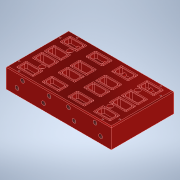
# Autodesk Inventor part: UNLHEP-14-01-P-004_ChuckForGantry
Saved by Autodesk Inventor 2022 (Build 260153000, 153)
## iProperties
Created: 2014-01-09
Part Number: UNLHEP-14-01-P-004_ChuckForGantry
Material: Aluminum, Anodized Red
Document SubType Name: Modeling
Designer: Frank Meier
Density: 2.7 g/cm^3
Project: UNL Pixel Phase I
Mass: 2699.72 g
Surface Area: 1115.91 cm^2
Volume: 999.896 cm^3
Appearance: Anodized - Red
Author: Frank Meier
Revision Number: 00
Autodesk Inventor part; units mm, degrees
ref_plane "YZ Plane" through (0, 0, 0) normal (1, 0, 0) x (0, 1, 0)
ref_plane "XZ Plane" through (0, 0, 0) normal (0, 1, 0) x (-1, 0, 0)
ref_plane "XY Plane" through (0, 0, 0) normal (0, 0, 1) x (1, 0, 0)
sketch "Skizze1" plane through (0, 0, 0) normal (0, 0, 1) x (1, 0, 0)
  line L0 (-117.475, -69.85) -> (117.475, -69.85)
  line L1 (117.475, -69.85) -> (117.475, 69.85)
  line L2 (117.475, 69.85) -> (-117.475, 69.85)
  line L3 (-117.475, 69.85) -> (-117.475, -69.85)
  line L4 (-117.475, -69.85) -> (117.475, 69.85) construction
  line L5 (117.475, -69.85) -> (-117.475, 69.85) construction
  point P0 (0, 0)
  dimension "d0" = 234.95
  dimension "d2" = 139.7
  constraints: 12 end point, 2 midpoint, 2 parallel, 1 horizontal, 1 perpendicular
  measures "d0" distance of L1.end L2.end
  measures "d2" distance of L0.end L1.end
extrude "Extrusion1" add sketch "Skizze1" along normal blind 44.45
chamfer "Fase1" distance 2 angle 45 4 edges at (0, -69.85, 44.45) (-117.475, 0, 44.45) (0, 69.85, 44.45) (117.475, 0, 44.45)
sketch "Alignment Holes" plane through (0, 0, 44.45) normal (0, 0, 1) x (1, 0, 0)
  line L0 (117.475, 69.85) -> (-117.475, 69.85) projected
  line L1 (117.475, -69.85) -> (117.475, 69.85) projected
  line L2 (-117.475, 69.85) -> (-117.475, -69.85) projected
  line L3 (-117.475, -69.85) -> (117.475, -69.85) projected
  point P0 (-112.475, 45.85)
  point P1 (-112.475, -45.85)
  point P2 (-93.475, -64.85)
  point P3 (-93.475, 64.85)
  point P4 (93.475, 64.85)
  point P5 (112.475, 45.85)
  point P6 (112.475, -45.85)
  point P7 (93.475, -64.85)
  dimension "d153" = 24
  dimension "d154" = 24
  dimension "d155" = 5
  dimension "d156" = 5
  dimension "d157" = 24
  dimension "d158" = 5
  dimension "d159" = 5
  dimension "d160" = 24
  dimension "d161" = 24
  dimension "d162" = 5
  dimension "d163" = 5
  dimension "d164" = 24
  dimension "d165" = 5
  dimension "d166" = 24
  dimension "d167" = 5
  dimension "d168" = 24
  measures "d153" distance from line of L0 point (-112.475, 45.85)
  measures "d154" distance from line of L3 point (-112.475, -45.85)
  measures "d155" distance from line of L2 point (-112.475, -45.85)
  measures "d156" distance from line of L3 point (-93.475, -64.85)
  measures "d157" distance from line of L2 point (-93.475, -64.85)
  measures "d158" distance from line of L2 point (-112.475, 45.85)
  measures "d159" distance from line of L0 point (-93.475, 64.85)
  measures "d160" distance from line of L2 point (-93.475, 64.85)
  measures "d161" distance from line of L1 point (93.475, 64.85)
  measures "d162" distance from line of L0 point (93.475, 64.85)
  measures "d163" distance from line of L1 point (112.475, 45.85)
  measures "d164" distance from line of L0 point (112.475, 45.85)
  measures "d165" distance from line of L1 point (112.475, -45.85)
  measures "d166" distance from line of L3 point (112.475, -45.85)
  measures "d167" distance from line of L3 point (93.475, -64.85)
  measures "d168" distance from line of L1 point (93.475, -64.85)
hole "Bohrung7" at (-112.475, 45.85, 44.45) at (-112.475, -45.85, 44.45) at (-93.475, -64.85, 44.45) at (-93.475, 64.85, 44.45) at (93.475, 64.85, 44.45) at (112.475, 45.85, 44.45) at (112.475, -45.85, 44.45) at (93.475, -64.85, 44.45) direction (0, 0, -1) diameter 3.242 depth 20 tip angle 118 thread size "M4x0.7" class "6H" standard "ISO Metric profile"
sketch "Wells" plane through (0, 0, 44.45) normal (0, 0, 1) x (1, 0, 0)
  line L0 (-97.975, 56.35) -> (-73.975, 56.35)
  line L1 (-70.975, 53.35) -> (-70.975, 44.35)
  line L2 (-73.975, 41.35) -> (-97.975, 41.35)
  line L3 (-100.975, 44.35) -> (-100.975, 53.35)
  circle A0 centre (-93.475, 64.85) radius 1.621 projected
  circle A1 centre (-112.475, 45.85) radius 1.621 projected
  arc A2 (-97.975, 56.35) -> (-100.975, 53.35) centre (-97.975, 53.35) ccw
  arc A3 (-70.975, 53.35) -> (-73.975, 56.35) centre (-73.975, 53.35) ccw
  arc A4 (-73.975, 41.35) -> (-70.975, 44.35) centre (-73.975, 44.35) ccw
  arc A5 (-100.975, 44.35) -> (-97.975, 41.35) centre (-97.975, 44.35) ccw
  arc A6 (-40.658, 56.35) -> (-43.658, 53.35) centre (-40.658, 53.35) ccw
  line L4 (-43.658, 44.35) -> (-43.658, 53.35)
  arc A7 (-43.658, 44.35) -> (-40.658, 41.35) centre (-40.658, 44.35) ccw
  line L5 (-40.658, 56.35) -> (-16.658, 56.35)
  arc A8 (-13.658, 53.35) -> (-16.658, 56.35) centre (-16.658, 53.35) ccw
  line L6 (-13.658, 53.35) -> (-13.658, 44.35)
  line L7 (-16.658, 41.35) -> (-40.658, 41.35)
  arc A9 (-16.658, 41.35) -> (-13.658, 44.35) centre (-16.658, 44.35) ccw
  arc A10 (16.659, 56.35) -> (13.659, 53.35) centre (16.659, 53.35) ccw
  line L8 (13.659, 44.35) -> (13.659, 53.35)
  arc A11 (13.659, 44.35) -> (16.659, 41.35) centre (16.659, 44.35) ccw
  line L9 (16.659, 56.35) -> (40.659, 56.35)
  arc A12 (43.659, 53.35) -> (40.659, 56.35) centre (40.659, 53.35) ccw
  line L10 (43.659, 53.35) -> (43.659, 44.35)
  line L11 (40.659, 41.35) -> (16.659, 41.35)
  arc A13 (40.659, 41.35) -> (43.659, 44.35) centre (40.659, 44.35) ccw
  arc A14 (73.976, 56.35) -> (70.976, 53.35) centre (73.976, 53.35) ccw
  line L12 (70.976, 44.35) -> (70.976, 53.35)
  arc A15 (70.976, 44.35) -> (73.976, 41.35) centre (73.976, 44.35) ccw
  line L13 (73.976, 56.35) -> (97.976, 56.35)
  arc A16 (100.976, 53.35) -> (97.976, 56.35) centre (97.976, 53.35) ccw
  line L14 (100.976, 53.35) -> (100.976, 44.35)
  line L15 (97.976, 41.35) -> (73.976, 41.35)
  arc A17 (97.976, 41.35) -> (100.976, 44.35) centre (97.976, 44.35) ccw
  arc A18 (-97.975, 20.784) -> (-100.975, 17.784) centre (-97.975, 17.784) ccw
  line L16 (-100.975, 8.784) -> (-100.975, 17.784)
  arc A19 (-100.975, 8.784) -> (-97.975, 5.784) centre (-97.975, 8.784) ccw
  line L17 (-97.975, 20.784) -> (-73.975, 20.784)
  arc A20 (-70.975, 17.784) -> (-73.975, 20.784) centre (-73.975, 17.784) ccw
  line L18 (-70.975, 17.784) -> (-70.975, 8.784)
  line L19 (-73.975, 5.784) -> (-97.975, 5.784)
  arc A21 (-73.975, 5.784) -> (-70.975, 8.784) centre (-73.975, 8.784) ccw
  arc A22 (-40.658, 20.784) -> (-43.658, 17.784) centre (-40.658, 17.784) ccw
  line L20 (-43.658, 8.784) -> (-43.658, 17.784)
  arc A23 (-43.658, 8.784) -> (-40.658, 5.784) centre (-40.658, 8.784) ccw
  line L21 (-40.658, 20.784) -> (-16.658, 20.784)
  arc A24 (-13.658, 17.784) -> (-16.658, 20.784) centre (-16.658, 17.784) ccw
  line L22 (-13.658, 17.784) -> (-13.658, 8.784)
  line L23 (-16.658, 5.784) -> (-40.658, 5.784)
  arc A25 (-16.658, 5.784) -> (-13.658, 8.784) centre (-16.658, 8.784) ccw
  arc A26 (16.659, 20.784) -> (13.659, 17.784) centre (16.659, 17.784) ccw
  line L24 (13.659, 8.784) -> (13.659, 17.784)
  arc A27 (13.659, 8.784) -> (16.659, 5.784) centre (16.659, 8.784) ccw
  line L25 (16.659, 20.784) -> (40.659, 20.784)
  arc A28 (43.659, 17.784) -> (40.659, 20.784) centre (40.659, 17.784) ccw
  line L26 (43.659, 17.784) -> (43.659, 8.784)
  line L27 (40.659, 5.784) -> (16.659, 5.784)
  arc A29 (40.659, 5.784) -> (43.659, 8.784) centre (40.659, 8.784) ccw
  arc A30 (73.976, 20.784) -> (70.976, 17.784) centre (73.976, 17.784) ccw
  line L28 (70.976, 8.784) -> (70.976, 17.784)
  arc A31 (70.976, 8.784) -> (73.976, 5.784) centre (73.976, 8.784) ccw
  line L29 (73.976, 20.784) -> (97.976, 20.784)
  arc A32 (100.976, 17.784) -> (97.976, 20.784) centre (97.976, 17.784) ccw
  line L30 (100.976, 17.784) -> (100.976, 8.784)
  line L31 (97.976, 5.784) -> (73.976, 5.784)
  arc A33 (97.976, 5.784) -> (100.976, 8.784) centre (97.976, 8.784) ccw
  circle A34 centre (-93.475, -64.85) radius 1.621 projected
  circle A35 centre (112.475, 45.85) radius 1.621 projected
  line L32 (97.975, -56.35) -> (73.975, -56.35)
  line L33 (70.975, -53.35) -> (70.975, -44.35)
  line L34 (73.975, -41.35) -> (97.975, -41.35)
  line L35 (100.975, -44.35) -> (100.975, -53.35)
  circle A36 centre (112.475, -45.85) radius 1.621 projected
  circle A37 centre (93.475, -64.85) radius 1.621 projected
  arc A38 (73.975, -41.35) -> (70.975, -44.35) centre (73.975, -44.35) ccw
  arc A39 (70.975, -53.35) -> (73.975, -56.35) centre (73.975, -53.35) ccw
  arc A40 (97.975, -56.35) -> (100.975, -53.35) centre (97.975, -53.35) ccw
  arc A41 (100.975, -44.35) -> (97.975, -41.35) centre (97.975, -44.35) ccw
  arc A42 (43.658, -44.35) -> (40.658, -41.35) centre (40.658, -44.35) ccw
  line L36 (16.658, -41.35) -> (40.658, -41.35)
  line L37 (43.658, -44.35) -> (43.658, -53.35)
  arc A43 (40.658, -56.35) -> (43.658, -53.35) centre (40.658, -53.35) ccw
  line L38 (40.658, -56.35) -> (16.658, -56.35)
  arc A44 (16.658, -41.35) -> (13.658, -44.35) centre (16.658, -44.35) ccw
  arc A45 (13.658, -53.35) -> (16.658, -56.35) centre (16.658, -53.35) ccw
  line L39 (13.658, -53.35) -> (13.658, -44.35)
  arc A46 (-13.659, -44.35) -> (-16.659, -41.35) centre (-16.659, -44.35) ccw
  line L40 (-40.659, -41.35) -> (-16.659, -41.35)
  line L41 (-13.659, -44.35) -> (-13.659, -53.35)
  arc A47 (-16.659, -56.35) -> (-13.659, -53.35) centre (-16.659, -53.35) ccw
  line L42 (-16.659, -56.35) -> (-40.659, -56.35)
  arc A48 (-40.659, -41.35) -> (-43.659, -44.35) centre (-40.659, -44.35) ccw
  arc A49 (-43.659, -53.35) -> (-40.659, -56.35) centre (-40.659, -53.35) ccw
  line L43 (-43.659, -53.35) -> (-43.659, -44.35)
  arc A50 (-70.976, -44.35) -> (-73.976, -41.35) centre (-73.976, -44.35) ccw
  line L44 (-97.976, -41.35) -> (-73.976, -41.35)
  line L45 (-70.976, -44.35) -> (-70.976, -53.35)
  arc A51 (-73.976, -56.35) -> (-70.976, -53.35) centre (-73.976, -53.35) ccw
  line L46 (-73.976, -56.35) -> (-97.976, -56.35)
  arc A52 (-97.976, -41.35) -> (-100.976, -44.35) centre (-97.976, -44.35) ccw
  arc A53 (-100.976, -53.35) -> (-97.976, -56.35) centre (-97.976, -53.35) ccw
  line L47 (-100.976, -53.35) -> (-100.976, -44.35)
  arc A54 (100.975, -8.784) -> (97.975, -5.784) centre (97.975, -8.784) ccw
  line L48 (73.975, -5.784) -> (97.975, -5.784)
  line L49 (100.975, -8.784) -> (100.975, -17.784)
  arc A55 (97.975, -20.784) -> (100.975, -17.784) centre (97.975, -17.784) ccw
  line L50 (97.975, -20.784) -> (73.975, -20.784)
  arc A56 (73.975, -5.784) -> (70.975, -8.784) centre (73.975, -8.784) ccw
  arc A57 (70.975, -17.784) -> (73.975, -20.784) centre (73.975, -17.784) ccw
  line L51 (70.975, -17.784) -> (70.975, -8.784)
  arc A58 (43.658, -8.784) -> (40.658, -5.784) centre (40.658, -8.784) ccw
  line L52 (16.658, -5.784) -> (40.658, -5.784)
  line L53 (43.658, -8.784) -> (43.658, -17.784)
  arc A59 (40.658, -20.784) -> (43.658, -17.784) centre (40.658, -17.784) ccw
  line L54 (40.658, -20.784) -> (16.658, -20.784)
  arc A60 (16.658, -5.784) -> (13.658, -8.784) centre (16.658, -8.784) ccw
  arc A61 (13.658, -17.784) -> (16.658, -20.784) centre (16.658, -17.784) ccw
  line L55 (13.658, -17.784) -> (13.658, -8.784)
  arc A62 (-13.659, -8.784) -> (-16.659, -5.784) centre (-16.659, -8.784) ccw
  line L56 (-40.659, -5.784) -> (-16.659, -5.784)
  line L57 (-13.659, -8.784) -> (-13.659, -17.784)
  arc A63 (-16.659, -20.784) -> (-13.659, -17.784) centre (-16.659, -17.784) ccw
  line L58 (-16.659, -20.784) -> (-40.659, -20.784)
  arc A64 (-40.659, -5.784) -> (-43.659, -8.784) centre (-40.659, -8.784) ccw
  arc A65 (-43.659, -17.784) -> (-40.659, -20.784) centre (-40.659, -17.784) ccw
  line L59 (-43.659, -17.784) -> (-43.659, -8.784)
  arc A66 (-70.976, -8.784) -> (-73.976, -5.784) centre (-73.976, -8.784) ccw
  line L60 (-97.976, -5.784) -> (-73.976, -5.784)
  line L61 (-70.976, -8.784) -> (-70.976, -17.784)
  arc A67 (-73.976, -20.784) -> (-70.976, -17.784) centre (-73.976, -17.784) ccw
  line L62 (-73.976, -20.784) -> (-97.976, -20.784)
  arc A68 (-97.976, -5.784) -> (-100.976, -8.784) centre (-97.976, -8.784) ccw
  arc A69 (-100.976, -17.784) -> (-97.976, -20.784) centre (-97.976, -17.784) ccw
  line L63 (-100.976, -17.784) -> (-100.976, -8.784)
  point P0 (0, 0)
  point P1 (-70.975, 41.35)
  point P2 (-70.975, 56.35)
  point P3 (-100.975, 41.35)
  point P4 (-43.658, 41.35)
  point P5 (-13.658, 56.35)
  point P6 (-13.658, 41.35)
  point P7 (13.659, 41.35)
  point P8 (43.659, 56.35)
  point P9 (43.659, 41.35)
  point P10 (70.976, 41.35)
  point P11 (100.976, 56.35)
  point P12 (100.976, 41.35)
  point P13 (-100.975, 5.784)
  point P14 (-70.975, 20.784)
  point P15 (-70.975, 5.784)
  point P16 (-43.658, 5.784)
  point P17 (-13.658, 20.784)
  point P18 (-13.658, 5.784)
  point P19 (13.659, 5.784)
  point P20 (43.659, 20.784)
  point P21 (43.659, 5.784)
  point P22 (70.976, 5.784)
  point P23 (100.976, 20.784)
  point P24 (100.976, 5.784)
  point P25 (100.975, -56.35)
  point P26 (70.975, -56.35)
  point P27 (100.975, -41.35)
  point P28 (43.658, -41.35)
  point P29 (43.658, -56.35)
  point P30 (13.658, -56.35)
  point P31 (-13.659, -41.35)
  point P32 (-13.659, -56.35)
  point P33 (-43.659, -56.35)
  point P34 (-70.976, -41.35)
  point P35 (-70.976, -56.35)
  point P36 (-100.976, -56.35)
  point P37 (100.975, -5.784)
  point P38 (100.975, -20.784)
  point P39 (70.975, -20.784)
  point P40 (43.658, -5.784)
  point P41 (43.658, -20.784)
  point P42 (13.658, -20.784)
  point P43 (-13.659, -5.784)
  point P44 (-13.659, -20.784)
  point P45 (-43.659, -20.784)
  point P46 (-70.976, -5.784)
  point P47 (-70.976, -20.784)
  point P48 (-100.976, -20.784)
  dimension "d259" = 30
  dimension "d260" = 15
  dimension "d261" = 8.5
  dimension "d262" = 11.5
  dimension "d266" = 3
  dimension "d269" = 57.317
  dimension "d272" = 35.566
  dimension "d276" = 11.499
  dimension "d410" = 11.5
  dimension "d411" = 8.5
  dimension "d412" = 15
  dimension "d413" = 30
  dimension "d414" = 3
  dimension "d417" = 57.317
  dimension "d420" = 35.566
  constraints: 128 end point, 128 point on circle, 96 point on line, 64 centre point, 16 tangent, 6 equal radius, 4 collinear, 4 horizontal, 4 parallel, 2 perpendicular, 2 vertical, 318 other
  measures "d259" distance of point (-70.975, 41.35) point (-100.975, 41.35)
  measures "d260" distance of point (-70.975, 56.35) point (-70.975, 41.35)
  measures "d261" distance from line of L0 A0.centre
  measures "d262" distance from line of L3 A1.centre
  measures "d266" radius of A2
  measures "d269" distance of L3.end L4.end
  measures "d272" distance of L3.end L16.end
  measures "d276" distance from line of L14 A35.centre
  measures "d410" distance from line of L35 A36.centre
  measures "d411" distance from line of A37.centre L32
  measures "d412" distance of point (100.975, -41.35) point (100.975, -56.35)
  measures "d413" distance of point (100.975, -56.35) point (70.975, -56.35)
  measures "d414" radius of A38
  measures "d417" distance of point (100.975, -41.35) point (43.658, -41.35)
  measures "d420" distance of point (100.975, -41.35) point (100.975, -5.784)
extrude "Extrusion6" cut sketch "Wells" against normal blind 10 contours L0 A3 L1 A4 L2 A5 L3 A2 | L5 A8 L6 A9 L7 A7 L4 A6 | L9 A12 L10 A13 L11 A11 L8 A10 | L13 A16 L14 A17 L15 A15 L12 A14 | L32 A39 L33 A38 L34 A41 L35 A40 | L37 A43 L38 A45 L39 A44 L36 A42 | L41 A47 L42 A49 L43 A48 L40 A46 | L45 A51 L46 A53 L47 A52 L44 A50
extrude "Extrusion7" cut sketch "Wells" against normal blind 30 contours L17 A20 L18 A21 L19 A19 L16 A18 | L21 A24 L22 A25 L23 A23 L20 A22 | L25 A28 L26 A29 L27 A27 L24 A26 | L29 A32 L30 A33 L31 A31 L28 A30 | L49 A55 L50 A57 L51 A56 L48 A54 | L53 A59 L54 A61 L55 A60 L52 A58 | L57 A63 L58 A65 L59 A64 L56 A62 | L61 A67 L62 A69 L63 A68 L60 A66
sketch "Sketch17" plane through (-117.475, -69.85, 0) normal (0, -1, 0) x (1, 0, 0)
  line L0 (232.95, 44.45) -> (2, 44.45) projected
  line L1 (46.499, 44.45) -> (46.499, 14.45) projected
  line L2 (188.45, 44.45) -> (188.45, 14.45) projected
  point P0 (117.475, 0)
  point P1 (36.499, 34.45)
  point P2 (23.999, 14.45)
  point P3 (83.316, 14.45)
  point P4 (95.816, 34.45)
  point P5 (198.45, 34.45)
  point P6 (210.95, 14.45)
  point P7 (139.133, 34.45)
  point P8 (151.633, 14.45)
  dimension "d283" = 10
  dimension "d286" = 59.317
  dimension "d328" = 59.317
  dimension "d443" = 10
  dimension "d444" = 10
  dimension "d450" = 20
  dimension "d451" = 12.5
  dimension "d452" = 12.5
  constraints: 2 horizontal, 2 horizontal alignment, 4 other
  measures "d283" distance from line of L0 point (36.499, 34.45)
  measures "d286" distance of point (23.999, 14.45) point (83.316, 14.45)
  measures "d328" distance of point (198.45, 34.45) point (139.133, 34.45)
  measures "d443" distance from line of L1 point (36.499, 34.45)
  measures "d444" distance from line of L2 point (198.45, 34.45)
  measures "d450" vertical distance of point (23.999, 14.45) point (36.499, 34.45)
  measures "d451" horizontal distance of point (23.999, 14.45) point (36.499, 34.45)
  measures "d452" horizontal distance of point (210.95, 14.45) point (198.45, 34.45)
hole "Hole12" at (-80.976, -69.85, 34.45) at (-21.659, -69.85, 34.45) at (21.658, -69.85, 34.45) at (80.975, -69.85, 34.45) direction (0, 1, 0) diameter 7.9502 depth 20 tip angle 118 taper from width 8.7366 to width 8.304 over 6.924 thread size "1/8" designation "1/8 - 27 NPT" standard "NPT"
hole "Hole13" at (-93.476, -69.85, 14.45) at (-34.159, -69.85, 14.45) at (34.158, -69.85, 14.45) at (93.475, -69.85, 14.45) direction (0, 1, 0) diameter 7.9502 depth 55 tip angle 118 taper from width 8.7366 to width 8.304 over 6.924 thread size "1/8" designation "1/8 - 27 NPT" standard "NPT"
sketch "Sketch19" plane through (-117.475, 69.85, 0) normal (0, 1, 0) x (1, 0, 0)
  arc A0 (40.4741, -34.45) -> (32.5239, -34.45) centre (36.499, -34.45) ccw projected
  circle A1 centre (95.816, -34.45) radius 3.9751 projected
  circle A2 centre (139.133, -34.45) radius 4.152 projected
  circle A3 centre (210.95, -14.45) radius 4.3684
  circle A4 centre (198.45, -34.45) radius 3.9751 projected
  line L0 (210.95, -23.476) -> (212.571, -24.45) projected
  line L1 (210.95, -23.476) -> (209.329, -24.45) projected
  point P0 (117.475, 0)
  point P1 (23.999, -14.5362)
  point P2 (83.316, -14.45)
  point P3 (95.816, -14.45)
  point P4 (151.633, -14.393)
  dimension "d446" = 12.5
  dimension "d447" = 12.5
  dimension "d448" = 12.5
  dimension "d449" = 12.5
  constraints: 5 coincident, 1 centre point, 1 vertical alignment
  measures "d446" horizontal distance of point (210.95, -14.45) point (198.45, -34.45)
  measures "d447" horizontal distance of point (151.633, -14.393) point (139.133, -34.45)
  measures "d448" horizontal distance of A1.centre point (83.316, -14.45)
  measures "d449" horizontal distance of point (23.999, -14.536) A0.centre
hole "Hole15" at (93.475, 69.85, 14.45) at (-34.159, 69.85, 14.45) at (-93.476, 69.85, 14.5362) at (34.158, 69.85, 14.393) direction (0, -1, 0) diameter 7.9502 depth 55 tip angle 118 taper from width 8.7366 to width 8.304 over 6.924 thread size "1/8" designation "1/8 - 27 NPT" standard "NPT"
hole "Hole16" at (-80.976, 69.85, 34.45) at (-21.659, 69.85, 34.45) at (21.658, 69.85, 34.45) at (80.975, 69.85, 34.45) direction (0, -1, 0) diameter 7.9502 depth 20 tip angle 118 taper from width 8.7366 to width 8.304 over 6.924 thread size "1/8" designation "1/8 - 27 NPT" standard "NPT"
sketch "Sketch22" plane through (0, 0, 44.45) normal (0, 0, 1) x (1, 0, 0)
  point P0 (0, 0)
  point P1 (76.2, -31)
  point P2 (-76.2, -31)
  point P3 (-76.2, 31)
  point P4 (76.2, 31)
  dimension "d382" = 76.2
  dimension "d383" = 152.4
  dimension "d384" = 31
  dimension "d385" = 62
  constraints: 2 horizontal alignment, 2 vertical alignment
  measures "d382" horizontal distance of point (76.2, -31) point (0, 0)
  measures "d383" distance of point (76.2, -31) point (-76.2, -31)
  measures "d384" vertical distance of point (76.2, -31) point (0, 0)
  measures "d385" distance of point (76.2, -31) point (76.2, 31)
hole "Hole18" at (76.2, -31, 44.45) at (-76.2, -31, 44.45) at (-76.2, 31, 44.45) at (76.2, 31, 44.45) direction (0, 0, -1) diameter 6.756 end through all counterbore diameter 11.113 counterbore depth 6.35 clearance for "Socket Head Cap Screw" size "1/4" standard "Ansi Unified Screw Threads"
sketch "Seal Seating" plane through (0, 0, 44.45) normal (0, 0, 1) x (1, 0, 0)
  line L0 (-71.475, 39.85) -> (-100.475, 39.85)
  line L1 (-102.475, 41.85) -> (-102.475, 55.85)
  line L2 (-100.475, 57.85) -> (-71.475, 57.85)
  line L3 (-69.475, 55.85) -> (-69.475, 41.85)
  line L4 (-97.975, 56.35) -> (-73.975, 56.35) projected
  line L5 (-70.975, 53.35) -> (-70.975, 44.35) projected
  line L6 (-100.975, 44.35) -> (-100.975, 53.35) projected
  line L7 (-73.975, 41.35) -> (-97.975, 41.35) projected
  line L8 (-69.0938, 37.4687) -> (-102.8562, 37.4687)
  line L9 (-104.8562, 39.4687) -> (-104.8563, 58.2313)
  line L10 (-102.8562, 60.2313) -> (-69.0938, 60.2313)
  line L11 (-67.0938, 58.2313) -> (-67.0938, 39.4687)
  arc A0 (-100.475, 57.85) -> (-102.475, 55.85) centre (-100.475, 55.85) ccw
  arc A1 (-102.475, 41.85) -> (-100.475, 39.85) centre (-100.475, 41.85) ccw
  arc A2 (-71.475, 39.85) -> (-69.475, 41.85) centre (-71.475, 41.85) ccw
  arc A3 (-69.475, 55.85) -> (-71.475, 57.85) centre (-71.475, 55.85) ccw
  arc A4 (-102.8562, 60.2313) -> (-104.8563, 58.2313) centre (-102.8562, 58.2313) ccw
  arc A5 (-104.8562, 39.4687) -> (-102.8562, 37.4687) centre (-102.8562, 39.4687) ccw
  arc A6 (-69.0938, 37.4687) -> (-67.0938, 39.4687) centre (-69.0938, 39.4687) ccw
  arc A7 (-67.0938, 58.2313) -> (-69.0938, 60.2313) centre (-69.0938, 58.2313) ccw
  line L12 (-14.158, 39.85) -> (-43.158, 39.85)
  line L13 (-11.7767, 37.4687) -> (-45.5392, 37.4687)
  line L14 (-45.5392, 60.2313) -> (-11.7767, 60.2313)
  line L15 (-43.158, 57.85) -> (-14.158, 57.85)
  line L16 (-12.158, 55.85) -> (-12.158, 41.85)
  line L17 (-45.158, 41.85) -> (-45.158, 55.85)
  arc A8 (-43.158, 57.85) -> (-45.158, 55.85) centre (-43.158, 55.85) ccw
  arc A9 (-45.5392, 60.2313) -> (-47.5392, 58.2313) centre (-45.5392, 58.2313) ccw
  line L18 (-47.5392, 39.4687) -> (-47.5392, 58.2313)
  arc A10 (-45.158, 41.85) -> (-43.158, 39.85) centre (-43.158, 41.85) ccw
  arc A11 (-47.5392, 39.4687) -> (-45.5392, 37.4687) centre (-45.5392, 39.4687) ccw
  arc A12 (-11.7767, 37.4687) -> (-9.7767, 39.4687) centre (-11.7767, 39.4687) ccw
  arc A13 (-9.7767, 58.2313) -> (-11.7767, 60.2313) centre (-11.7767, 58.2313) ccw
  arc A14 (-14.158, 39.85) -> (-12.158, 41.85) centre (-14.158, 41.85) ccw
  line L19 (-9.7767, 58.2313) -> (-9.7767, 39.4687)
  arc A15 (-12.158, 55.85) -> (-14.158, 57.85) centre (-14.158, 55.85) ccw
  line L20 (43.159, 39.85) -> (14.159, 39.85)
  line L21 (45.5403, 37.4687) -> (11.7778, 37.4687)
  line L22 (11.7778, 60.2313) -> (45.5403, 60.2313)
  line L23 (14.159, 57.85) -> (43.159, 57.85)
  line L24 (45.159, 55.85) -> (45.159, 41.85)
  line L25 (12.159, 41.85) -> (12.159, 55.85)
  arc A16 (14.159, 57.85) -> (12.159, 55.85) centre (14.159, 55.85) ccw
  arc A17 (11.7778, 60.2313) -> (9.7778, 58.2313) centre (11.7778, 58.2313) ccw
  line L26 (9.7778, 39.4687) -> (9.7778, 58.2313)
  arc A18 (12.159, 41.85) -> (14.159, 39.85) centre (14.159, 41.85) ccw
  arc A19 (9.7778, 39.4687) -> (11.7778, 37.4687) centre (11.7778, 39.4687) ccw
  arc A20 (45.5403, 37.4687) -> (47.5403, 39.4687) centre (45.5403, 39.4687) ccw
  arc A21 (47.5403, 58.2313) -> (45.5403, 60.2313) centre (45.5403, 58.2313) ccw
  arc A22 (43.159, 39.85) -> (45.159, 41.85) centre (43.159, 41.85) ccw
  line L27 (47.5403, 58.2313) -> (47.5403, 39.4687)
  arc A23 (45.159, 55.85) -> (43.159, 57.85) centre (43.159, 55.85) ccw
  line L28 (100.476, 39.85) -> (71.476, 39.85)
  line L29 (102.8573, 37.4688) -> (69.0948, 37.4688)
  line L30 (69.0948, 60.2313) -> (102.8573, 60.2313)
  line L31 (71.476, 57.85) -> (100.476, 57.85)
  line L32 (102.476, 55.85) -> (102.476, 41.85)
  line L33 (69.476, 41.85) -> (69.476, 55.85)
  arc A24 (71.476, 57.85) -> (69.476, 55.85) centre (71.476, 55.85) ccw
  arc A25 (69.0948, 60.2313) -> (67.0948, 58.2313) centre (69.0948, 58.2313) ccw
  line L34 (67.0948, 39.4688) -> (67.0948, 58.2313)
  arc A26 (69.476, 41.85) -> (71.476, 39.85) centre (71.476, 41.85) ccw
  arc A27 (67.0948, 39.4688) -> (69.0948, 37.4688) centre (69.0948, 39.4688) ccw
  arc A28 (102.8573, 37.4688) -> (104.8573, 39.4688) centre (102.8573, 39.4688) ccw
  arc A29 (104.8573, 58.2313) -> (102.8573, 60.2313) centre (102.8573, 58.2313) ccw
  arc A30 (100.476, 39.85) -> (102.476, 41.85) centre (100.476, 41.85) ccw
  line L35 (104.8573, 58.2313) -> (104.8573, 39.4688)
  arc A31 (102.476, 55.85) -> (100.476, 57.85) centre (100.476, 55.85) ccw
  line L36 (-71.475, 4.284) -> (-100.475, 4.284)
  line L37 (-69.0938, 1.9027) -> (-102.8562, 1.9027)
  line L38 (-102.8562, 24.6653) -> (-69.0938, 24.6653)
  line L39 (-100.475, 22.284) -> (-71.475, 22.284)
  line L40 (-69.475, 20.284) -> (-69.475, 6.284)
  line L41 (-102.475, 6.284) -> (-102.475, 20.284)
  arc A32 (-100.475, 22.284) -> (-102.475, 20.284) centre (-100.475, 20.284) ccw
  arc A33 (-102.8562, 24.6653) -> (-104.8563, 22.6652) centre (-102.8562, 22.6652) ccw
  line L42 (-104.8562, 3.9027) -> (-104.8563, 22.6652)
  arc A34 (-102.475, 6.284) -> (-100.475, 4.284) centre (-100.475, 6.284) ccw
  arc A35 (-104.8562, 3.9027) -> (-102.8562, 1.9027) centre (-102.8562, 3.9027) ccw
  arc A36 (-69.0938, 1.9027) -> (-67.0937, 3.9027) centre (-69.0938, 3.9027) ccw
  arc A37 (-67.0937, 22.6653) -> (-69.0938, 24.6653) centre (-69.0938, 22.6653) ccw
  arc A38 (-71.475, 4.284) -> (-69.475, 6.284) centre (-71.475, 6.284) ccw
  line L43 (-67.0937, 22.6653) -> (-67.0937, 3.9027)
  arc A39 (-69.475, 20.284) -> (-71.475, 22.284) centre (-71.475, 20.284) ccw
  line L44 (-14.158, 4.284) -> (-43.158, 4.284)
  line L45 (-11.7767, 1.9027) -> (-45.5392, 1.9027)
  line L46 (-45.5392, 24.6653) -> (-11.7767, 24.6653)
  line L47 (-43.158, 22.284) -> (-14.158, 22.284)
  line L48 (-12.158, 20.284) -> (-12.158, 6.284)
  line L49 (-45.158, 6.284) -> (-45.158, 20.284)
  arc A40 (-43.158, 22.284) -> (-45.158, 20.284) centre (-43.158, 20.284) ccw
  arc A41 (-45.5392, 24.6653) -> (-47.5392, 22.6653) centre (-45.5392, 22.6653) ccw
  line L50 (-47.5392, 3.9027) -> (-47.5392, 22.6653)
  arc A42 (-45.158, 6.284) -> (-43.158, 4.284) centre (-43.158, 6.284) ccw
  arc A43 (-47.5392, 3.9027) -> (-45.5392, 1.9027) centre (-45.5392, 3.9027) ccw
  arc A44 (-11.7767, 1.9027) -> (-9.7767, 3.9027) centre (-11.7767, 3.9027) ccw
  arc A45 (-9.7767, 22.6653) -> (-11.7767, 24.6653) centre (-11.7767, 22.6653) ccw
  arc A46 (-14.158, 4.284) -> (-12.158, 6.284) centre (-14.158, 6.284) ccw
  line L51 (-9.7767, 22.6653) -> (-9.7767, 3.9027)
  arc A47 (-12.158, 20.284) -> (-14.158, 22.284) centre (-14.158, 20.284) ccw
  line L52 (43.159, 4.284) -> (14.159, 4.284)
  line L53 (45.5403, 1.9027) -> (11.7778, 1.9027)
  line L54 (11.7778, 24.6653) -> (45.5403, 24.6653)
  line L55 (14.159, 22.284) -> (43.159, 22.284)
  line L56 (45.159, 20.284) -> (45.159, 6.284)
  line L57 (12.159, 6.284) -> (12.159, 20.284)
  arc A48 (14.159, 22.284) -> (12.159, 20.284) centre (14.159, 20.284) ccw
  arc A49 (11.7778, 24.6653) -> (9.7778, 22.6653) centre (11.7778, 22.6653) ccw
  line L58 (9.7778, 3.9027) -> (9.7778, 22.6653)
  arc A50 (12.159, 6.284) -> (14.159, 4.284) centre (14.159, 6.284) ccw
  arc A51 (9.7778, 3.9027) -> (11.7778, 1.9027) centre (11.7778, 3.9027) ccw
  arc A52 (45.5403, 1.9027) -> (47.5403, 3.9027) centre (45.5403, 3.9027) ccw
  arc A53 (47.5403, 22.6653) -> (45.5403, 24.6653) centre (45.5403, 22.6653) ccw
  arc A54 (43.159, 4.284) -> (45.159, 6.284) centre (43.159, 6.284) ccw
  line L59 (47.5403, 22.6653) -> (47.5403, 3.9027)
  arc A55 (45.159, 20.284) -> (43.159, 22.284) centre (43.159, 20.284) ccw
  line L60 (100.476, 4.284) -> (71.476, 4.284)
  line L61 (102.8573, 1.9028) -> (69.0948, 1.9028)
  line L62 (69.0948, 24.6653) -> (102.8573, 24.6653)
  line L63 (71.476, 22.284) -> (100.476, 22.284)
  line L64 (102.476, 20.284) -> (102.476, 6.284)
  line L65 (69.476, 6.284) -> (69.476, 20.284)
  arc A56 (71.476, 22.284) -> (69.476, 20.284) centre (71.476, 20.284) ccw
  arc A57 (69.0948, 24.6653) -> (67.0948, 22.6653) centre (69.0948, 22.6653) ccw
  line L66 (67.0948, 3.9027) -> (67.0948, 22.6653)
  arc A58 (69.476, 6.284) -> (71.476, 4.284) centre (71.476, 6.284) ccw
  arc A59 (67.0948, 3.9027) -> (69.0948, 1.9028) centre (69.0948, 3.9027) ccw
  arc A60 (102.8573, 1.9028) -> (104.8573, 3.9028) centre (102.8573, 3.9028) ccw
  arc A61 (104.8573, 22.6653) -> (102.8573, 24.6653) centre (102.8573, 22.6653) ccw
  arc A62 (100.476, 4.284) -> (102.476, 6.284) centre (100.476, 6.284) ccw
  line L67 (104.8573, 22.6653) -> (104.8573, 3.9028)
  arc A63 (102.476, 20.284) -> (100.476, 22.284) centre (100.476, 20.284) ccw
  line L68 (-71.476, -57.85) -> (-100.476, -57.85)
  line L69 (-102.476, -55.85) -> (-102.476, -41.85)
  line L70 (-100.476, -39.85) -> (-71.476, -39.85)
  line L71 (-69.476, -41.85) -> (-69.476, -55.85)
  line L72 (-70.976, -44.35) -> (-70.976, -53.35) projected
  line L73 (-97.976, -41.35) -> (-73.976, -41.35) projected
  line L74 (-100.976, -53.35) -> (-100.976, -44.35) projected
  line L75 (-73.976, -56.35) -> (-97.976, -56.35) projected
  arc A64 (-100.476, -39.85) -> (-102.476, -41.85) centre (-100.476, -41.85) ccw
  arc A65 (-102.476, -55.85) -> (-100.476, -57.85) centre (-100.476, -55.85) ccw
  arc A66 (-71.476, -57.85) -> (-69.476, -55.85) centre (-71.476, -55.85) ccw
  arc A67 (-69.476, -41.85) -> (-71.476, -39.85) centre (-71.476, -41.85) ccw
  line L76 (-69.0947, -60.2313) -> (-102.8573, -60.2313)
  line L77 (-104.8573, -58.2313) -> (-104.8573, -39.4688)
  line L78 (-102.8573, -37.4688) -> (-69.0947, -37.4688)
  line L79 (-67.0948, -39.4688) -> (-67.0948, -58.2313)
  arc A68 (-102.8573, -37.4688) -> (-104.8573, -39.4688) centre (-102.8573, -39.4688) ccw
  arc A69 (-104.8573, -58.2313) -> (-102.8573, -60.2313) centre (-102.8573, -58.2313) ccw
  arc A70 (-69.0947, -60.2313) -> (-67.0948, -58.2313) centre (-69.0947, -58.2313) ccw
  arc A71 (-67.0948, -39.4688) -> (-69.0947, -37.4688) centre (-69.0947, -39.4688) ccw
  line L80 (-14.159, -57.85) -> (-43.159, -57.85)
  line L81 (-45.159, -55.85) -> (-45.159, -41.85)
  line L82 (-43.159, -39.85) -> (-14.159, -39.85)
  line L83 (-11.7777, -60.2313) -> (-45.5403, -60.2313)
  line L84 (-45.5403, -37.4688) -> (-11.7777, -37.4688)
  line L85 (-12.159, -41.85) -> (-12.159, -55.85)
  arc A72 (-14.159, -57.85) -> (-12.159, -55.85) centre (-14.159, -55.85) ccw
  arc A73 (-11.7777, -60.2313) -> (-9.7777, -58.2313) centre (-11.7777, -58.2313) ccw
  line L86 (-9.7777, -39.4688) -> (-9.7777, -58.2313)
  arc A74 (-12.159, -41.85) -> (-14.159, -39.85) centre (-14.159, -41.85) ccw
  arc A75 (-9.7777, -39.4688) -> (-11.7777, -37.4688) centre (-11.7777, -39.4688) ccw
  arc A76 (-43.159, -39.85) -> (-45.159, -41.85) centre (-43.159, -41.85) ccw
  arc A77 (-45.5403, -37.4688) -> (-47.5403, -39.4688) centre (-45.5403, -39.4688) ccw
  line L87 (-47.5403, -58.2313) -> (-47.5403, -39.4688)
  arc A78 (-45.159, -55.85) -> (-43.159, -57.85) centre (-43.159, -55.85) ccw
  arc A79 (-47.5403, -58.2313) -> (-45.5403, -60.2313) centre (-45.5403, -58.2313) ccw
  line L88 (43.158, -57.85) -> (14.158, -57.85)
  line L89 (12.158, -55.85) -> (12.158, -41.85)
  line L90 (14.158, -39.85) -> (43.158, -39.85)
  line L91 (45.5393, -60.2313) -> (11.7767, -60.2313)
  line L92 (11.7767, -37.4688) -> (45.5393, -37.4688)
  line L93 (45.158, -41.85) -> (45.158, -55.85)
  arc A80 (43.158, -57.85) -> (45.158, -55.85) centre (43.158, -55.85) ccw
  arc A81 (45.5393, -60.2313) -> (47.5393, -58.2313) centre (45.5393, -58.2313) ccw
  line L94 (47.5393, -39.4688) -> (47.5393, -58.2313)
  arc A82 (45.158, -41.85) -> (43.158, -39.85) centre (43.158, -41.85) ccw
  arc A83 (47.5393, -39.4688) -> (45.5393, -37.4688) centre (45.5393, -39.4688) ccw
  arc A84 (14.158, -39.85) -> (12.158, -41.85) centre (14.158, -41.85) ccw
  arc A85 (11.7767, -37.4688) -> (9.7767, -39.4688) centre (11.7767, -39.4688) ccw
  line L95 (9.7767, -58.2313) -> (9.7767, -39.4688)
  arc A86 (12.158, -55.85) -> (14.158, -57.85) centre (14.158, -55.85) ccw
  arc A87 (9.7767, -58.2313) -> (11.7767, -60.2313) centre (11.7767, -58.2313) ccw
  line L96 (100.475, -57.85) -> (71.475, -57.85)
  line L97 (69.475, -55.85) -> (69.475, -41.85)
  line L98 (71.475, -39.85) -> (100.475, -39.85)
  line L99 (102.8562, -60.2312) -> (69.0937, -60.2312)
  line L100 (69.0937, -37.4687) -> (102.8562, -37.4687)
  line L101 (102.475, -41.85) -> (102.475, -55.85)
  arc A88 (100.475, -57.85) -> (102.475, -55.85) centre (100.475, -55.85) ccw
  arc A89 (102.8562, -60.2312) -> (104.8563, -58.2313) centre (102.8562, -58.2313) ccw
  line L102 (104.8563, -39.4687) -> (104.8563, -58.2313)
  arc A90 (102.475, -41.85) -> (100.475, -39.85) centre (100.475, -41.85) ccw
  arc A91 (104.8563, -39.4687) -> (102.8562, -37.4687) centre (102.8562, -39.4687) ccw
  arc A92 (71.475, -39.85) -> (69.475, -41.85) centre (71.475, -41.85) ccw
  arc A93 (69.0937, -37.4687) -> (67.0938, -39.4687) centre (69.0937, -39.4687) ccw
  line L103 (67.0937, -58.2313) -> (67.0938, -39.4687)
  arc A94 (69.475, -55.85) -> (71.475, -57.85) centre (71.475, -55.85) ccw
  arc A95 (67.0937, -58.2313) -> (69.0937, -60.2312) centre (69.0937, -58.2313) ccw
  line L104 (-71.476, -22.284) -> (-100.476, -22.284)
  line L105 (-102.476, -20.284) -> (-102.476, -6.284)
  line L106 (-100.476, -4.284) -> (-71.476, -4.284)
  line L107 (-69.0948, -24.6653) -> (-102.8573, -24.6653)
  line L108 (-102.8573, -1.9028) -> (-69.0948, -1.9028)
  line L109 (-69.476, -6.284) -> (-69.476, -20.284)
  arc A96 (-71.476, -22.284) -> (-69.476, -20.284) centre (-71.476, -20.284) ccw
  arc A97 (-69.0948, -24.6653) -> (-67.0948, -22.6653) centre (-69.0948, -22.6653) ccw
  line L110 (-67.0948, -3.9028) -> (-67.0948, -22.6653)
  arc A98 (-69.476, -6.284) -> (-71.476, -4.284) centre (-71.476, -6.284) ccw
  arc A99 (-67.0948, -3.9028) -> (-69.0948, -1.9028) centre (-69.0948, -3.9028) ccw
  arc A100 (-100.476, -4.284) -> (-102.476, -6.284) centre (-100.476, -6.284) ccw
  arc A101 (-102.8573, -1.9028) -> (-104.8573, -3.9028) centre (-102.8573, -3.9028) ccw
  line L111 (-104.8573, -22.6653) -> (-104.8573, -3.9028)
  arc A102 (-102.476, -20.284) -> (-100.476, -22.284) centre (-100.476, -20.284) ccw
  arc A103 (-104.8573, -22.6653) -> (-102.8573, -24.6653) centre (-102.8573, -22.6653) ccw
  line L112 (-14.159, -22.284) -> (-43.159, -22.284)
  line L113 (-45.159, -20.284) -> (-45.159, -6.284)
  line L114 (-43.159, -4.284) -> (-14.159, -4.284)
  line L115 (-11.7778, -24.6653) -> (-45.5403, -24.6653)
  line L116 (-45.5403, -1.9028) -> (-11.7778, -1.9028)
  line L117 (-12.159, -6.284) -> (-12.159, -20.284)
  arc A104 (-14.159, -22.284) -> (-12.159, -20.284) centre (-14.159, -20.284) ccw
  arc A105 (-11.7778, -24.6653) -> (-9.7777, -22.6653) centre (-11.7778, -22.6653) ccw
  line L118 (-9.7777, -3.9028) -> (-9.7777, -22.6653)
  arc A106 (-12.159, -6.284) -> (-14.159, -4.284) centre (-14.159, -6.284) ccw
  arc A107 (-9.7777, -3.9028) -> (-11.7778, -1.9028) centre (-11.7778, -3.9028) ccw
  arc A108 (-43.159, -4.284) -> (-45.159, -6.284) centre (-43.159, -6.284) ccw
  arc A109 (-45.5403, -1.9028) -> (-47.5403, -3.9028) centre (-45.5403, -3.9028) ccw
  line L119 (-47.5403, -22.6653) -> (-47.5403, -3.9028)
  arc A110 (-45.159, -20.284) -> (-43.159, -22.284) centre (-43.159, -20.284) ccw
  arc A111 (-47.5403, -22.6653) -> (-45.5403, -24.6653) centre (-45.5403, -22.6653) ccw
  line L120 (43.158, -22.284) -> (14.158, -22.284)
  line L121 (12.158, -20.284) -> (12.158, -6.284)
  line L122 (14.158, -4.284) -> (43.158, -4.284)
  line L123 (45.5392, -24.6653) -> (11.7767, -24.6653)
  line L124 (11.7767, -1.9027) -> (45.5392, -1.9027)
  line L125 (45.158, -6.284) -> (45.158, -20.284)
  arc A112 (43.158, -22.284) -> (45.158, -20.284) centre (43.158, -20.284) ccw
  arc A113 (45.5392, -24.6653) -> (47.5393, -22.6653) centre (45.5392, -22.6653) ccw
  line L126 (47.5393, -3.9027) -> (47.5393, -22.6653)
  arc A114 (45.158, -6.284) -> (43.158, -4.284) centre (43.158, -6.284) ccw
  arc A115 (47.5393, -3.9027) -> (45.5392, -1.9027) centre (45.5392, -3.9027) ccw
  arc A116 (14.158, -4.284) -> (12.158, -6.284) centre (14.158, -6.284) ccw
  arc A117 (11.7767, -1.9027) -> (9.7767, -3.9028) centre (11.7767, -3.9028) ccw
  line L127 (9.7767, -22.6653) -> (9.7767, -3.9028)
  arc A118 (12.158, -20.284) -> (14.158, -22.284) centre (14.158, -20.284) ccw
  arc A119 (9.7767, -22.6653) -> (11.7767, -24.6653) centre (11.7767, -22.6653) ccw
  line L128 (100.475, -22.284) -> (71.475, -22.284)
  line L129 (69.475, -20.284) -> (69.475, -6.284)
  line L130 (71.475, -4.284) -> (100.475, -4.284)
  line L131 (102.8562, -24.6652) -> (69.0937, -24.6652)
  line L132 (69.0937, -1.9027) -> (102.8562, -1.9027)
  line L133 (102.475, -6.284) -> (102.475, -20.284)
  arc A120 (100.475, -22.284) -> (102.475, -20.284) centre (100.475, -20.284) ccw
  arc A121 (102.8562, -24.6652) -> (104.8563, -22.6652) centre (102.8562, -22.6652) ccw
  line L134 (104.8563, -3.9027) -> (104.8563, -22.6652)
  arc A122 (102.475, -6.284) -> (100.475, -4.284) centre (100.475, -6.284) ccw
  arc A123 (104.8563, -3.9027) -> (102.8562, -1.9027) centre (102.8562, -3.9027) ccw
  arc A124 (71.475, -4.284) -> (69.475, -6.284) centre (71.475, -6.284) ccw
  arc A125 (69.0937, -1.9027) -> (67.0937, -3.9027) centre (69.0937, -3.9027) ccw
  line L135 (67.0937, -22.6652) -> (67.0937, -3.9027)
  arc A126 (69.475, -20.284) -> (71.475, -22.284) centre (71.475, -20.284) ccw
  arc A127 (67.0937, -22.6652) -> (69.0937, -24.6652) centre (69.0937, -22.6652) ccw
  point P0 (0, 0)
  dimension "d393" = 1.5
  dimension "d394" = 1.5
  dimension "d395" = 1.5
  dimension "d396" = 1.5
  dimension "d397" = 2.3813
  dimension "d398" = 2.3813
  dimension "d399" = 2.3813
  dimension "d400" = 2.3813
  dimension "d401" = 2
  dimension "d404" = 57.317
  dimension "d407" = 35.566
  dimension "d423" = 1.5
  dimension "d424" = 1.5
  dimension "d425" = 1.5
  dimension "d426" = 1.5
  dimension "d427" = 2
  dimension "d428" = 2.3813
  dimension "d429" = 2.3813
  dimension "d430" = 2.3813
  dimension "d431" = 2.3813
  dimension "d432" = 2
  dimension "d435" = 57.317
  dimension "d438" = 35.566
  constraints: 256 end point, 256 point on circle, 128 centre point, 32 tangent, 13 equal radius, 8 parallel, 6 horizontal, 4 collinear, 4 perpendicular, 2 vertical, 556 other
  measures "d393" distance between parallel lines of L2 L4
  measures "d394" distance between parallel lines of L3 L5
  measures "d395" distance between parallel lines of L6 L1
  measures "d396" distance between parallel lines of L0 L7
  measures "d397" distance between parallel lines of L2 L10
  measures "d398" distance between parallel lines of L3 L11
  measures "d399" distance between parallel lines of L8 L0
  measures "d400" distance between parallel lines of L9 L1
  measures "d401" radius of A0
  measures "d404" distance of L0.start L12.start
  measures "d407" distance of L0.start L36.start
  measures "d423" distance between parallel lines of L72 L71
  measures "d424" distance between parallel lines of L70 L73
  measures "d425" distance between parallel lines of L69 L74
  measures "d426" distance between parallel lines of L75 L68
  measures "d427" radius of A64
  measures "d428" distance between parallel lines of L78 L70
  measures "d429" distance between parallel lines of L71 L79
  measures "d430" distance between parallel lines of L76 L68
  measures "d431" distance between parallel lines of L77 L69
  measures "d432" radius of A68
  measures "d435" distance of L78.end L84.end
  measures "d438" distance of L78.end L108.end
extrude "Extrusion9" cut sketch "Seal Seating" against normal blind 2.3813
equation "\"d328\" = d286"
